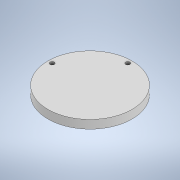
# Autodesk Inventor part: drum
Saved by Autodesk Inventor 2022 (Build 260153000, 153)
## iProperties
Created: 2022-05-21
Part Number: drum
Material: Generic
Document SubType Name: Modeling
Designer: kylem
Density: 1 g/cm^3
Appearance: Default
Author: kylem
Autodesk Inventor part; units mm, degrees
ref_plane "YZ Plane" through (0, 0, 0) normal (1, 0, 0) x (0, 1, 0)
ref_plane "XZ Plane" through (0, 0, 0) normal (0, 1, 0) x (-1, 0, 0)
ref_plane "XY Plane" through (0, 0, 0) normal (0, 0, 1) x (1, 0, 0)
sketch "Sketch1" plane through (0, 0, 0) normal (0, 1, 0) x (-1, 0, 0)
  circle A0 centre (0, 0) radius 10
  line L0 (0, 0) -> (10, 0)
  line L1 (0, 0) -> (0, -10)
  line L2 (10, 0) -> (9, 0)
  line L3 (0, -10) -> (0, -9)
  circle A1 centre (9, 0) radius 0.5
  circle A2 centre (0, -9) radius 0.5
  dimension "d0" = 20
  dimension "d1" = 1
  dimension "d2" = 1
  dimension "d3" = 1
  dimension "d4" = 1
  constraints: 8 end point, 3 centre point, 3 coincident, 2 point on circle, 2 point on line, 1 horizontal, 1 perpendicular
  measures "d0" diameter of A0
  measures "d1" distance of L0.end L2.end
  measures "d2" distance of L1.end L3.end
  measures "d3" diameter of A1
  measures "d4" diameter of A2
extrude "Extrusion1" add sketch "Sketch1" along normal blind 2 contours L0 A1 L1 A2 A0 | A0 L1 A2 L0 A1
body "Solid1"
